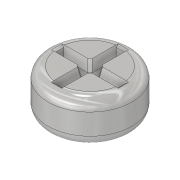
# Autodesk Inventor part: Kepala Baut
Saved by Autodesk Inventor 2019 (Build 230136000, 136)
## iProperties
Created: 2021-10-16
Part Number: Kepala Baut
Material: Generic
Document SubType Name: Modeling
Designer: user
Density: 1 g/cm^3
Appearance: Polished - Small Pyramid Knurl
Author: user
Autodesk Inventor part; units mm, degrees
ref_plane "YZ Plane" through (0, 0, 0) normal (1, 0, 0) x (0, 1, 0)
ref_plane "XZ Plane" through (0, 0, 0) normal (0, 1, 0) x (-1, 0, 0)
ref_plane "XY Plane" through (0, 0, 0) normal (0, 0, 1) x (1, 0, 0)
sketch "Sketch1" plane through (0, 0, 0) normal (0, 1, 0) x (-1, 0, 0)
  circle A0 centre (0, 0) radius 2
  dimension "d0" = 4
  constraints: 1 centre point, 1 coincident
  measures "d0" diameter of A0
extrude "Extrusion1" add sketch "Sketch1" along normal blind 2
fillet "Fillet1" radius 0.5 2 edges at (2, 2, 0) (2, 0, 0)
sketch "Sketch2" plane through (0, 2, 0) normal (0, 1, 0) x (1, 0, 0)
  line L0 (0.25, 1.5) -> (-0.25, 1.5)
  line L1 (-0.25, -1.5) -> (0.25, -1.5)
  line L2 (0.25, -1.5) -> (-0.25, 1.5) construction
  line L3 (0.25, 1.5) -> (-0.25, -1.5) construction
  line L4 (0.25, 1.5) -> (-0.25, 1.5)
  line L5 (-0.25, -1.5) -> (0.25, -1.5)
  line L6 (0.25, -1.5) -> (-0.25, 1.5) construction
  line L7 (0.25, 1.5) -> (-0.25, -1.5) construction
  line L8 (1.5, -0.25) -> (1.5, 0.25)
  line L9 (-1.5, 0.25) -> (-1.5, -0.25)
  line L10 (-1.5, -0.25) -> (1.5, 0.25) construction
  line L11 (1.5, -0.25) -> (-1.5, 0.25) construction
  line L12 (1.5, -0.25) -> (1.5, 0.25)
  line L13 (-1.5, 0.25) -> (-1.5, -0.25)
  line L14 (-1.5, -0.25) -> (1.5, 0.25) construction
  line L15 (1.5, -0.25) -> (-1.5, 0.25) construction
  line L16 (-0.25, 1.5) -> (-0.25, 0.25)
  line L17 (-0.25, -0.25) -> (-0.25, -1.5)
  line L18 (-1.5, -0.25) -> (-0.25, -0.25)
  line L19 (0.25, -0.25) -> (1.5, -0.25)
  line L20 (0.25, -1.5) -> (0.25, -0.25)
  line L21 (0.25, 0.25) -> (0.25, 1.5)
  line L22 (1.5, 0.25) -> (0.25, 0.25)
  line L23 (-0.25, 0.25) -> (-1.5, 0.25)
  line L24 (-1.5, -0.25) -> (-0.25, -0.25)
  line L25 (0.25, -0.25) -> (1.5, -0.25)
  line L26 (0.25, -1.5) -> (0.25, -0.25)
  line L27 (0.25, 0.25) -> (0.25, 1.5)
  line L28 (1.5, 0.25) -> (0.25, 0.25)
  line L29 (-0.25, 0.25) -> (-1.5, 0.25)
  line L30 (-0.25, 1.5) -> (-0.25, 0.25)
  line L31 (-0.25, -0.25) -> (-0.25, -1.5)
  point P0 (0, 0)
  point P1 (0, 0)
  dimension "d5" = 0.5
  dimension "d8" = 3
  dimension "d9" = 0.5
  dimension "d10" = 3
  constraints: 64 end point, 20 parallel, 8 perpendicular
  measures "d5" distance of L0.end L0.start
  measures "d8" distance of L9.start L8.end
  measures "d9" distance of L8.end L8.start
  measures "d10" distance of L13.start L12.end
extrude "Extrusion2" cut sketch "Sketch2" against normal blind 0.5 draft -10
chamfer "Chamfer1" distance 0.1 angle 45 12 edges at (-1.5, 2, 0.1259) (-1.5, 2, -0.1259) (-0.2059, 1.75, 0.2059) (-0.2059, 1.75, -0.2059) (0.2059, 1.75, -0.2059) (0.2059, 1.75, 0.2059) (0.1259, 2, -1.5) (-0.1259, 2, -1.5) (1.5, 2, 0.1259) (1.5, 2, -0.1259) (-0.1259, 2, 1.5) (0.1259, 2, 1.5)
body "Solid1"
